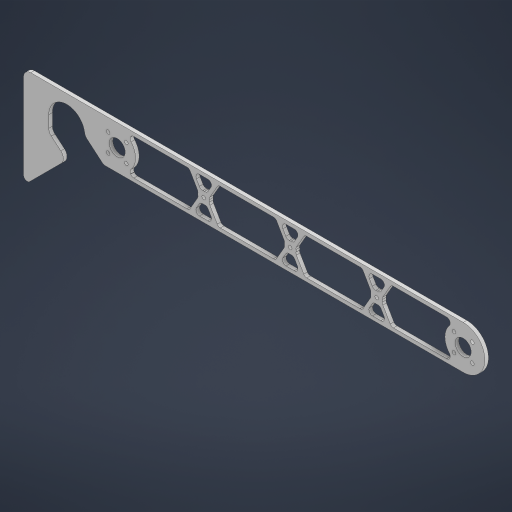
# Autodesk Inventor part: Arm1stLink
Saved by Autodesk Inventor 2023 (Build 270158000, 158)
## iProperties
Created: 2023-12-24
Part Number: Arm1stLink
Material: Generic
Document SubType Name: Modeling
Designer: kelle
Density: 1 g/cm^3
Appearance: Default
Author: kelle
Autodesk Inventor part; units mm, degrees
ref_plane "YZ Plane" through (0, 0, 0) normal (1, 0, 0) x (0, 1, 0)
ref_plane "XZ Plane" through (0, 0, 0) normal (0, 1, 0) x (-1, 0, 0)
ref_plane "XY Plane" through (0, 0, 0) normal (0, 0, 1) x (1, 0, 0)
sketch "Sketch1" plane through (0, 0, 0) normal (0, 0, 1) x (1, 0, 0)
  line L0 (152.4, 0) -> (-152.4, 0) construction
  line L1 (152.4, 19.05) -> (-152.4, 19.05)
  line L2 (-152.4, -19.05) -> (152.4, -19.05)
  arc A0 (152.4, -19.05) -> (152.4, 19.05) centre (152.4, 0) ccw
  arc A1 (-152.4, 19.05) -> (-152.4, -19.05) centre (-152.4, 0) ccw
  circle A2 centre (-152.4, 0) radius 7
  line L3 (-160.4, -8) -> (-144.4, -8) construction
  line L4 (-144.4, -8) -> (-144.4, 8) construction
  line L5 (-144.4, 8) -> (-160.4, 8) construction
  line L6 (-160.4, 8) -> (-160.4, -8) construction
  line L7 (-160.4, -8) -> (-144.4, 8) construction
  line L8 (-144.4, -8) -> (-160.4, 8) construction
  circle A3 centre (-160.4, 8) radius 1.5875
  circle A4 centre (-144.4, 8) radius 1.5875
  circle A5 centre (-160.4, -8) radius 1.5875
  circle A6 centre (-144.4, -8) radius 1.5875
  line L9 (0, 19.05) -> (0, -19.05) construction
  line L10 (-152.4, 0) -> (152.4, 0) construction
  circle A7 centre (152.4, 0) radius 7
  line L11 (160.4, -8) -> (144.4, -8) construction
  line L12 (144.4, -8) -> (144.4, 8) construction
  line L13 (144.4, 8) -> (160.4, 8) construction
  line L14 (160.4, 8) -> (160.4, -8) construction
  line L15 (160.4, -8) -> (144.4, 8) construction
  line L16 (144.4, -8) -> (160.4, 8) construction
  circle A8 centre (160.4, 8) radius 1.5875
  circle A9 centre (144.4, 8) radius 1.5875
  circle A10 centre (160.4, -8) radius 1.5875
  circle A11 centre (144.4, -8) radius 1.5875
  circle A12 centre (0, 0) radius 2
  circle A13 centre (-76.2, 0) radius 2
  circle A14 centre (76.2, 0) radius 2
  circle A15 centre (0, 0) radius 2
  dimension "d0" = 152.4
  dimension "d1" = 38.1
  dimension "d2" = 14
  dimension "d3" = 16
  dimension "d4" = 16
  dimension "d5" = 3.175
  dimension "d8" = 16
  dimension "d11" = 16
  dimension "d14" = 4
  dimension "d17" = 76.2
  dimension "d20" = 76.2
  constraints: 38 end point, 16 centre point, 11 symmetric about line, 5 coincident, 5 horizontal, 5 midpoint, 4 point on circle, 4 tangent, 3 parallel, 1 perpendicular, 1 vertical, 17 other
  measures "d0" distance of point (0, 0) L0.end
  measures "d1" diameter of A1
  measures "d2" diameter of A2
  measures "d3" distance of L5.end L4.end
  measures "d4" distance of L4.end L3.end
  measures "d5" diameter of A3
  measures "d8" distance of A3.centre A4.centre
  measures "d11" distance of A3.centre A5.centre
  measures "d14" diameter of A12
  measures "d17" distance of A12.centre A13.centre
  measures "d20" distance of A12.centre A14.centre
extrude "Extrusion1" add sketch "Sketch1" along normal blind 3.175
sketch "Sketch2" plane through (0, 0, 3.175) normal (0, 0, 1) x (1, 0, 0)
  arc A0 (-152.4, 19.05) -> (-152.4, -19.05) centre (-152.4, 0) ccw projected
  line L0 (-152.4, -19.05) -> (152.4, -19.05) projected
  arc A1 (152.4, -19.05) -> (152.4, 19.05) centre (152.4, 0) ccw projected
  line L1 (152.4, 19.05) -> (-152.4, 19.05) construction
  circle A2 centre (0, 0) radius 2 projected
  circle A3 centre (-76.2, 0) radius 2 projected
  circle A4 centre (76.2, 0) radius 2 projected
  circle A5 centre (160.4, -8) radius 1.5875 projected
  circle A6 centre (160.4, 8) radius 1.5875 projected
  circle A7 centre (152.4, 0) radius 7 projected
  circle A8 centre (144.4, -8) radius 1.5875 projected
  circle A9 centre (144.4, 8) radius 1.5875 projected
  circle A10 centre (-144.4, -8) radius 1.5875 projected
  circle A11 centre (-160.4, -8) radius 1.5875 projected
  circle A12 centre (-144.4, 8) radius 1.5875 projected
  circle A13 centre (-160.4, 8) radius 1.5875 projected
  circle A14 centre (-152.4, 0) radius 7 projected
  circle A15 centre (-152.4, 0) radius 12.9012 construction
  circle A16 centre (-152.4, 0) radius 16.0762
  arc A17 (-152.4, 15.875) -> (-152.4, -15.875) centre (-152.4, 0) ccw
  line L2 (-152.4, -15.875) -> (152.4, -15.875)
  arc A18 (152.4, -15.875) -> (152.4, 15.875) centre (152.4, 0) ccw
  line L3 (152.4, 15.875) -> (-152.4, 15.875)
  line L4 (-76.2, 19.05) -> (-76.2, -19.05) construction
  line L5 (-152.4, -19.05) -> (152.4, -19.05) construction
  line L6 (0, 19.05) -> (0, -19.05) construction
  circle A19 centre (152.4, 0) radius 16.0762
  circle A20 centre (-76.2, 0) radius 5.175
  circle A21 centre (0, 0) radius 5.175
  circle A22 centre (76.2, 0) radius 5.175
  line L7 (-152.4, 0) -> (-114.3, 0) construction
  line L8 (-152.4, 0) -> (-133.35, 32.9956)
  line L9 (-133.35, 32.9956) -> (-95.25, 32.9956)
  line L10 (-95.25, 32.9956) -> (-76.2, 0)
  line L11 (-76.2, 0) -> (-95.25, -32.9956)
  line L12 (-95.25, -32.9956) -> (-133.35, -32.9956)
  line L13 (-133.35, -32.9956) -> (-152.4, 0)
  line L14 (-97.0831, 29.8206) -> (-131.5169, 29.8206)
  line L15 (-131.5169, 29.8206) -> (-148.7338, 0)
  line L16 (-148.7338, 0) -> (-131.5169, -29.8206)
  line L17 (-131.5169, -29.8206) -> (-97.0831, -29.8206)
  line L18 (-97.0831, -29.8206) -> (-79.8662, 0)
  line L19 (-79.8662, 0) -> (-97.0831, 29.8206)
  line L20 (0, 0) -> (-19.05, 32.9956)
  line L21 (-57.15, 32.9956) -> (-76.2, 0)
  line L22 (-76.2, 0) -> (-57.15, -32.9956)
  line L23 (-19.05, -32.9956) -> (0, 0)
  line L24 (-20.8831, 29.8206) -> (-3.6662, 0)
  line L25 (-3.6662, 0) -> (-20.8831, -29.8206)
  line L26 (-55.3169, -29.8206) -> (-72.5338, 0)
  line L27 (-72.5338, 0) -> (-55.3169, 29.8206)
  line L28 (-152.4, 19.05) -> (152.4, 19.05)
  line L29 (152.4, 0) -> (133.35, 32.9956)
  line L30 (95.25, 32.9956) -> (76.2, 0)
  line L31 (76.2, 0) -> (95.25, -32.9956)
  line L32 (133.35, -32.9956) -> (152.4, 0)
  line L33 (131.5169, 29.8206) -> (148.7338, 0)
  line L34 (148.7338, 0) -> (131.5169, -29.8206)
  line L35 (97.0831, -29.8206) -> (79.8662, 0)
  line L36 (79.8662, 0) -> (97.0831, 29.8206)
  line L37 (20.8831, 29.8206) -> (3.6662, 0)
  line L38 (0, 0) -> (19.05, 32.9956)
  line L39 (19.05, -32.9956) -> (0, 0)
  line L40 (3.6662, 0) -> (20.8831, -29.8206)
  line L41 (55.3169, -29.8206) -> (72.5338, 0)
  line L42 (76.2, 0) -> (57.15, -32.9956)
  line L43 (72.5338, 0) -> (55.3169, 29.8206)
  line L44 (57.15, 32.9956) -> (76.2, 0)
  point P0 (141.7706, 12.0607)
  point P1 (139.5684, 15.875)
  point P2 (89.0316, 15.875)
  point P3 (80.9929, 1.9516)
  point P4 (80.9929, -1.9516)
  point P5 (89.0316, -15.875)
  point P6 (139.5684, -15.875)
  point P7 (141.7706, -12.0607)
  point P8 (85.3654, -15.875)
  point P9 (78.7875, -4.4817)
  point P10 (73.6125, -4.4817)
  point P11 (67.0346, -15.875)
  point P12 (78.7875, 4.4817)
  point P13 (85.3654, 15.875)
  point P14 (67.0346, 15.875)
  point P15 (73.6125, 4.4817)
  point P16 (12.8316, 15.875)
  point P17 (4.7929, 1.9516)
  point P18 (4.7929, -1.9516)
  point P19 (12.8316, -15.875)
  point P20 (63.3684, -15.875)
  point P21 (71.4071, -1.9516)
  point P22 (71.4071, 1.9516)
  point P23 (63.3684, 15.875)
  point P24 (9.1654, -15.875)
  point P25 (2.5875, -4.4817)
  point P26 (-2.5875, -4.4817)
  point P27 (-9.1654, -15.875)
  point P28 (2.5875, 4.4817)
  point P29 (9.1654, 15.875)
  point P30 (-9.1654, 15.875)
  point P31 (-2.5875, 4.4817)
  point P32 (-63.3684, 15.875)
  point P33 (-71.4071, 1.9516)
  point P34 (-71.4071, -1.9516)
  point P35 (-63.3684, -15.875)
  point P36 (-12.8316, -15.875)
  point P37 (-4.7929, -1.9516)
  point P38 (-4.7929, 1.9516)
  point P39 (-12.8316, 15.875)
  point P40 (-67.0346, -15.875)
  point P41 (-73.6125, -4.4817)
  point P42 (-78.7875, -4.4817)
  point P43 (-85.3654, -15.875)
  point P44 (-73.6125, 4.4817)
  point P45 (-67.0346, 15.875)
  point P46 (-85.3654, 15.875)
  point P47 (-78.7875, 4.4817)
  point P48 (-80.9929, 1.9516)
  point P49 (-89.0316, 15.875)
  point P50 (-139.5684, 15.875)
  point P51 (-141.7706, 12.0607)
  point P52 (-141.7706, -12.0607)
  point P53 (-139.5684, -15.875)
  point P54 (-89.0316, -15.875)
  point P55 (-80.9929, -1.9516)
  dimension "d25" = 3.175
  dimension "d26" = 3.175
  dimension "d27" = 3.175
  dimension "d28" = 3.175
  dimension "d29" = 3.175
  dimension "d30" = 38.1
  dimension "d31" = 3.175
  constraints: 84 end point, 36 symmetric about line, 8 centre point, 4 point on circle, 2 coincident, 2 midpoint, 2 point on line, 1 horizontal, 1 tangent, 1 vertical, 22 other
  measures "d25" radial gap between concentric circles of A15 A16
  measures "d26" distance between parallel lines of L1 L3
  measures "d27" radial gap between concentric circles of A3 A20
  measures "d28" radial gap between concentric circles of A2 A21
  measures "d29" radial gap between concentric circles of A4 A22
  measures "d30" distance of L7.start L7.end
  measures "d31" distance between parallel lines of L9 L14
extrude "Extrusion2" cut sketch "Sketch2" against normal through all contours L3 L19 A20 L18 L2 L16 A16 L15 | L3 L21 A20 L10 | L11 A20 L22 L2 | L3 L24 A21 L25 L2 L26 A20 L27 | L3 L38 A21 L20 | L23 A21 L39 L2 | L3 L43 A22 L41 L2 L40 A21 L37 | L3 L30 A22 L44 | L42 A22 L31 L2 | L3 L33 A19 L34 L2 L35 A22 L36
fillet "Fillet1" radius 3.175 56 edges at (-73.6125, -4.4817, 1.5875) (-67.0346, -15.875, 1.5875) (-78.7875, -4.4817, 1.5875) (-85.3654, -15.875, 1.5875) (2.5875, -4.4817, 1.5875) (9.1654, -15.875, 1.5875) (-2.5875, -4.4817, 1.5875) (-9.1654, -15.875, 1.5875) (-89.0316, 15.875, 1.5875) (-80.9929, 1.9516, 1.5875) (-139.5684, 15.875, 1.5875) (-141.7706, 12.0607, 1.5875) (-141.7706, -12.0607, 1.5875) (-139.5684, -15.875, 1.5875) (-89.0316, -15.875, 1.5875) (-80.9929, -1.9516, 1.5875) (78.7875, -4.4817, 1.5875) (85.3654, -15.875, 1.5875) (73.6125, -4.4817, 1.5875) (67.0346, -15.875, 1.5875) (4.7929, 1.9516, 1.5875) (12.8316, 15.875, 1.5875) (4.7929, -1.9516, 1.5875) (12.8316, -15.875, 1.5875) (63.3684, -15.875, 1.5875) (71.4071, -1.9516, 1.5875) (71.4071, 1.9516, 1.5875) (63.3684, 15.875, 1.5875) (139.5684, 15.875, 1.5875) (141.7706, 12.0607, 1.5875) (89.0316, 15.875, 1.5875) (80.9929, 1.9516, 1.5875) (80.9929, -1.9516, 1.5875) (89.0316, -15.875, 1.5875) (139.5684, -15.875, 1.5875) (141.7706, -12.0607, 1.5875) (-71.4071, 1.9516, 1.5875) (-63.3684, 15.875, 1.5875) (-71.4071, -1.9516, 1.5875) (-63.3684, -15.875, 1.5875) (-12.8316, -15.875, 1.5875) (-4.7929, -1.9516, 1.5875) (-4.7929, 1.9516, 1.5875) (-12.8316, 15.875, 1.5875) (-67.0346, 15.875, 1.5875) (-73.6125, 4.4817, 1.5875) (-85.3654, 15.875, 1.5875) (-78.7875, 4.4817, 1.5875) (9.1654, 15.875, 1.5875) (2.5875, 4.4817, 1.5875) (-9.1654, 15.875, 1.5875) (-2.5875, 4.4817, 1.5875) (85.3654, 15.875, 1.5875) (78.7875, 4.4817, 1.5875) (67.0346, 15.875, 1.5875) (73.6125, 4.4817, 1.5875)
sketch "Sketch3" plane through (0, 0, 3.175) normal (0, 0, 1) x (1, 0, 0)
  line L0 (-82.6158, -11.1125) -> (-80.0614, -6.6882) projected
  arc A0 (-76.889, -5.1289) -> (-80.0614, -6.6882) centre (-77.3118, -8.2757) ccw projected
  arc A1 (-76.889, -5.1289) -> (-75.511, -5.1289) centre (-76.2, 0) ccw projected
  arc A2 (-72.3386, -6.6882) -> (-75.511, -5.1289) centre (-75.0882, -8.2757) ccw projected
  line L1 (-72.3386, -6.6882) -> (-69.7842, -11.1125) projected
  arc A3 (-72.5338, -15.875) -> (-69.7842, -11.1125) centre (-72.5338, -12.7) ccw projected
  line L2 (-72.5338, -15.875) -> (-79.8662, -15.875) projected
  arc A4 (-82.6158, -11.1125) -> (-79.8662, -15.875) centre (-79.8662, -12.7) ccw projected
  line L3 (11.9151, -14.2875) -> (5.4607, -3.1082) projected
  arc A5 (5.0885, -0.9425) -> (5.4607, -3.1082) centre (8.2103, -1.5207) ccw projected
  arc A6 (5.0885, -0.9425) -> (5.0885, 0.9425) centre (0, 0) ccw projected
  arc A7 (5.4607, 3.1082) -> (5.0885, 0.9425) centre (8.2103, 1.5207) ccw projected
  line L4 (5.4607, 3.1082) -> (11.9151, 14.2875) projected
  arc A8 (14.6647, 15.875) -> (11.9151, 14.2875) centre (14.6647, 12.7) ccw projected
  line L5 (14.6647, 15.875) -> (61.5353, 15.875) projected
  arc A9 (64.2849, 14.2875) -> (61.5353, 15.875) centre (61.5353, 12.7) ccw projected
  line L6 (64.2849, 14.2875) -> (70.7393, 3.1082) projected
  arc A10 (71.1115, 0.9425) -> (70.7393, 3.1082) centre (67.9897, 1.5207) ccw projected
  arc A11 (71.1115, 0.9425) -> (71.1115, -0.9425) centre (76.2, 0) ccw projected
  arc A12 (70.7393, -3.1082) -> (71.1115, -0.9425) centre (67.9897, -1.5207) ccw projected
  line L7 (70.7393, -3.1082) -> (64.2849, -14.2875) projected
  arc A13 (61.5353, -15.875) -> (64.2849, -14.2875) centre (61.5353, -12.7) ccw projected
  line L8 (61.5353, -15.875) -> (14.6647, -15.875) projected
  arc A14 (11.9151, -14.2875) -> (14.6647, -15.875) centre (14.6647, -12.7) ccw projected
  line L9 (81.6607, 3.1082) -> (88.1151, 14.2875) projected
  arc A15 (90.8647, 15.875) -> (88.1151, 14.2875) centre (90.8647, 12.7) ccw projected
  line L10 (90.8647, 15.875) -> (137.7353, 15.875) projected
  arc A16 (140.4849, 14.2875) -> (137.7353, 15.875) centre (137.7353, 12.7) ccw projected
  line L11 (140.4849, 14.2875) -> (140.5635, 14.1515) projected
  arc A17 (140.2195, 10.4919) -> (140.5635, 14.1515) centre (137.8138, 12.564) ccw projected
  arc A18 (140.2195, 10.4919) -> (140.2195, -10.4919) centre (152.4, 0) ccw projected
  arc A19 (140.5635, -14.1515) -> (140.2195, -10.4919) centre (137.8138, -12.564) ccw projected
  line L12 (140.5635, -14.1515) -> (140.4849, -14.2875) projected
  arc A20 (137.7353, -15.875) -> (140.4849, -14.2875) centre (137.7353, -12.7) ccw projected
  line L13 (137.7353, -15.875) -> (90.8647, -15.875) projected
  arc A21 (88.1151, -14.2875) -> (90.8647, -15.875) centre (90.8647, -12.7) ccw projected
  line L14 (88.1151, -14.2875) -> (81.6607, -3.1082) projected
  arc A22 (81.2885, -0.9425) -> (81.6607, -3.1082) centre (84.4103, -1.5207) ccw projected
  arc A23 (81.2885, -0.9425) -> (81.2885, 0.9425) centre (76.2, 0) ccw projected
  arc A24 (81.6607, 3.1082) -> (81.2885, 0.9425) centre (84.4103, 1.5207) ccw projected
  line L15 (-6.4158, -11.1125) -> (-3.8614, -6.6882) projected
  arc A25 (-0.689, -5.1289) -> (-3.8614, -6.6882) centre (-1.1118, -8.2757) ccw projected
  arc A26 (-0.689, -5.1289) -> (0.689, -5.1289) centre (0, 0) ccw projected
  arc A27 (3.8614, -6.6882) -> (0.689, -5.1289) centre (1.1118, -8.2757) ccw projected
  line L16 (3.8614, -6.6882) -> (6.4158, -11.1125) projected
  arc A28 (3.6662, -15.875) -> (6.4158, -11.1125) centre (3.6662, -12.7) ccw projected
  line L17 (3.6662, -15.875) -> (-3.6662, -15.875) projected
  arc A29 (-6.4158, -11.1125) -> (-3.6662, -15.875) centre (-3.6662, -12.7) ccw projected
  line L18 (-80.0614, 6.6882) -> (-82.6158, 11.1125) projected
  arc A30 (-79.8662, 15.875) -> (-82.6158, 11.1125) centre (-79.8662, 12.7) ccw projected
  line L19 (-79.8662, 15.875) -> (-72.5338, 15.875) projected
  arc A31 (-69.7842, 11.1125) -> (-72.5338, 15.875) centre (-72.5338, 12.7) ccw projected
  line L20 (-69.7842, 11.1125) -> (-72.3386, 6.6882) projected
  arc A32 (-75.511, 5.1289) -> (-72.3386, 6.6882) centre (-75.0882, 8.2757) ccw projected
  arc A33 (-75.511, 5.1289) -> (-76.889, 5.1289) centre (-76.2, 0) ccw projected
  arc A34 (-80.0614, 6.6882) -> (-76.889, 5.1289) centre (-77.3118, 8.2757) ccw projected
  line L21 (-64.2849, -14.2875) -> (-70.7393, -3.1082) projected
  arc A35 (-71.1115, -0.9425) -> (-70.7393, -3.1082) centre (-67.9897, -1.5207) ccw projected
  arc A36 (-71.1115, -0.9425) -> (-71.1115, 0.9425) centre (-76.2, 0) ccw projected
  arc A37 (-70.7393, 3.1082) -> (-71.1115, 0.9425) centre (-67.9897, 1.5207) ccw projected
  line L22 (-70.7393, 3.1082) -> (-64.2849, 14.2875) projected
  arc A38 (-61.5353, 15.875) -> (-64.2849, 14.2875) centre (-61.5353, 12.7) ccw projected
  line L23 (-61.5353, 15.875) -> (-14.6647, 15.875) projected
  arc A39 (-11.9151, 14.2875) -> (-14.6647, 15.875) centre (-14.6647, 12.7) ccw projected
  line L24 (-11.9151, 14.2875) -> (-5.4607, 3.1082) projected
  arc A40 (-5.0885, 0.9425) -> (-5.4607, 3.1082) centre (-8.2103, 1.5207) ccw projected
  arc A41 (-5.0885, 0.9425) -> (-5.0885, -0.9425) centre (0, 0) ccw projected
  arc A42 (-5.4607, -3.1082) -> (-5.0885, -0.9425) centre (-8.2103, -1.5207) ccw projected
  line L25 (-5.4607, -3.1082) -> (-11.9151, -14.2875) projected
  arc A43 (-14.6647, -15.875) -> (-11.9151, -14.2875) centre (-14.6647, -12.7) ccw projected
  line L26 (-14.6647, -15.875) -> (-61.5353, -15.875) projected
  arc A44 (-64.2849, -14.2875) -> (-61.5353, -15.875) centre (-61.5353, -12.7) ccw projected
  line L27 (72.3386, 6.6882) -> (69.7842, 11.1125) projected
  arc A45 (72.5338, 15.875) -> (69.7842, 11.1125) centre (72.5338, 12.7) ccw projected
  line L28 (72.5338, 15.875) -> (79.8662, 15.875) projected
  arc A46 (82.6158, 11.1125) -> (79.8662, 15.875) centre (79.8662, 12.7) ccw projected
  line L29 (82.6158, 11.1125) -> (80.0614, 6.6882) projected
  arc A47 (76.889, 5.1289) -> (80.0614, 6.6882) centre (77.3118, 8.2757) ccw projected
  arc A48 (76.889, 5.1289) -> (75.511, 5.1289) centre (76.2, 0) ccw projected
  arc A49 (72.3386, 6.6882) -> (75.511, 5.1289) centre (75.0882, 8.2757) ccw projected
  line L30 (69.7842, -11.1125) -> (72.3386, -6.6882) projected
  arc A50 (75.511, -5.1289) -> (72.3386, -6.6882) centre (75.0882, -8.2757) ccw projected
  arc A51 (75.511, -5.1289) -> (76.889, -5.1289) centre (76.2, 0) ccw projected
  arc A52 (80.0614, -6.6882) -> (76.889, -5.1289) centre (77.3118, -8.2757) ccw projected
  line L31 (80.0614, -6.6882) -> (82.6158, -11.1125) projected
  arc A53 (79.8662, -15.875) -> (82.6158, -11.1125) centre (79.8662, -12.7) ccw projected
  line L32 (79.8662, -15.875) -> (72.5338, -15.875) projected
  arc A54 (69.7842, -11.1125) -> (72.5338, -15.875) centre (72.5338, -12.7) ccw projected
  line L33 (-3.8614, 6.6882) -> (-6.4158, 11.1125) projected
  arc A55 (-3.6662, 15.875) -> (-6.4158, 11.1125) centre (-3.6662, 12.7) ccw projected
  line L34 (-3.6662, 15.875) -> (3.6662, 15.875) projected
  arc A56 (6.4158, 11.1125) -> (3.6662, 15.875) centre (3.6662, 12.7) ccw projected
  line L35 (6.4158, 11.1125) -> (3.8614, 6.6882) projected
  arc A57 (0.689, 5.1289) -> (3.8614, 6.6882) centre (1.1118, 8.2757) ccw projected
  arc A58 (0.689, 5.1289) -> (-0.689, 5.1289) centre (0, 0) ccw projected
  arc A59 (-3.8614, 6.6882) -> (-0.689, 5.1289) centre (-1.1118, 8.2757) ccw projected
  line L36 (-140.5635, 14.1515) -> (-140.4849, 14.2875) projected
  arc A60 (-137.7353, 15.875) -> (-140.4849, 14.2875) centre (-137.7353, 12.7) ccw projected
  line L37 (-137.7353, 15.875) -> (-90.8647, 15.875) projected
  arc A61 (-88.1151, 14.2875) -> (-90.8647, 15.875) centre (-90.8647, 12.7) ccw projected
  line L38 (-88.1151, 14.2875) -> (-81.6607, 3.1082) projected
  arc A62 (-81.2885, 0.9425) -> (-81.6607, 3.1082) centre (-84.4103, 1.5207) ccw projected
  arc A63 (-81.2885, 0.9425) -> (-81.2885, -0.9425) centre (-76.2, 0) ccw projected
  arc A64 (-81.6607, -3.1082) -> (-81.2885, -0.9425) centre (-84.4103, -1.5207) ccw projected
  line L39 (-81.6607, -3.1082) -> (-88.1151, -14.2875) projected
  arc A65 (-90.8647, -15.875) -> (-88.1151, -14.2875) centre (-90.8647, -12.7) ccw projected
  line L40 (-90.8647, -15.875) -> (-137.7353, -15.875) projected
  arc A66 (-140.4849, -14.2875) -> (-137.7353, -15.875) centre (-137.7353, -12.7) ccw projected
  line L41 (-140.4849, -14.2875) -> (-140.5635, -14.1515) projected
  arc A67 (-140.2195, -10.4919) -> (-140.5635, -14.1515) centre (-137.8138, -12.564) ccw projected
  arc A68 (-140.2195, -10.4919) -> (-140.2195, 10.4919) centre (-152.4, 0) ccw projected
  arc A69 (-140.5635, 14.1515) -> (-140.2195, 10.4919) centre (-137.8138, 12.564) ccw projected
  arc A70 (-152.4, 19.05) -> (-152.4, -19.05) centre (-152.4, 0) ccw projected
  line L42 (-152.4, -19.05) -> (152.4, -19.05) projected
  arc A71 (152.4, -19.05) -> (152.4, 19.05) centre (152.4, 0) ccw projected
  line L43 (152.4, 19.05) -> (-152.4, 19.05) projected
  circle A72 centre (0, 0) radius 2 projected
  circle A73 centre (-76.2, 0) radius 2 projected
  circle A74 centre (76.2, 0) radius 2 projected
  circle A75 centre (160.4, -8) radius 1.5875 projected
  circle A76 centre (160.4, 8) radius 1.5875 projected
  circle A77 centre (152.4, 0) radius 7 projected
  circle A78 centre (144.4, -8) radius 1.5875 projected
  circle A79 centre (144.4, 8) radius 1.5875 projected
  circle A80 centre (-144.4, -8) radius 1.5875 projected
  circle A81 centre (-160.4, -8) radius 1.5875 projected
  circle A82 centre (-144.4, 8) radius 1.5875 projected
  circle A83 centre (-160.4, 8) radius 1.5875 projected
  circle A84 centre (-152.4, 0) radius 7 projected
  circle A85 centre (-76.2, 0) radius 2 projected
  circle A86 centre (-76.2, 0) radius 1.5875
  circle A87 centre (0, 0) radius 2 projected
  circle A88 centre (0, 0) radius 1.5875
  circle A89 centre (76.2, 0) radius 2 projected
  circle A90 centre (76.2, 0) radius 1.5875
  dimension "d35" = 3.175
  dimension "d36" = 3.175
  dimension "d37" = 3.175
  constraints: 3 centre point, 3 coincident
  measures "d35" diameter of A86
  measures "d36" diameter of A88
  measures "d37" diameter of A90
extrude "Extrusion3" add sketch "Sketch3" against normal blind 3.175 contours A72 | A73 | A74
sketch "Sketch4" plane through (0, 0, 3.175) normal (0, 0, 1) x (1, 0, 0)
  line L0 (152.4, 19.05) -> (-152.4, 19.05) projected
  line L1 (-152.4, 19.05) -> (-234.95, 19.05)
  line L2 (-234.95, 19.05) -> (-234.95, -19.05)
  line L3 (-234.95, -19.05) -> (-152.4, -19.05)
  line L4 (-152.4, -19.05) -> (-152.4, 19.05)
  line L5 (-234.95, 19.05) -> (-196.85, 19.05)
  line L6 (-196.85, 19.05) -> (-196.85, -69.85)
  line L7 (-196.85, -69.85) -> (-234.95, -69.85)
  line L8 (-234.95, -69.85) -> (-234.95, 19.05)
  line L9 (-234.95, -69.85) -> (-196.85, -31.75)
  circle A0 centre (-196.85, -5.0447) radius 15.875
  line L10 (-164.4274, -19.05) -> (-180.975, -5.0447)
  line L11 (-212.725, 0) -> (-212.725, -19.05)
  line L12 (-196.85, -31.75) -> (-212.725, -18.314)
  circle A1 centre (-152.4, 0) radius 7 projected
  circle A2 centre (-144.4, -8) radius 1.5875 projected
  circle A3 centre (-144.4, 8) radius 1.5875 projected
  circle A4 centre (-160.4, 8) radius 1.5875 projected
  circle A5 centre (-160.4, -8) radius 1.5875 projected
  point P0 (0, 0)
  point P1 (-211.8554, -19.05)
  point P2 (-212.725, -5.0447)
  point P3 (-152.4, -7)
  point P4 (-152.4, 7)
  dimension "d45" = 31.75
  dimension "d40" = 82.55
  dimension "d41" = 38.1
  dimension "d42" = 38.1
  dimension "d43" = 88.9
  dimension "d44" = 45
  constraints: 24 end point, 5 parallel, 5 point on line, 3 perpendicular, 2 horizontal, 1 vertical, 3 other
  measures "d40" distance of L3.end L2.end
  measures "d41" distance of L2.end L1.end
  measures "d42" distance of L6.end L7.end
  measures "d43" distance of L5.end L6.end
  measures "d44" angle of L7 L9
extrude "Extrusion4" add sketch "Sketch4" against normal blind 3.175 contours L4 A1 L3 L10 A0 L6 L1 | L6 A0 L11 L3 L2 L1 | L3 L12 L9 L8
fillet "Fillet2" radius 6.35 3 edges at (-211.8554, -19.05, 1.5875) (-212.725, -19.05, 1.5875) (-196.85, -31.75, 1.5875)
fillet "Fillet3" radius 6.35 2 edges at (-180.975, -5.0447, 1.5875) (-234.95, 19.05, 1.5875)
fillet "Fillet4" radius 3.175 2 edges at (-164.4274, -19.05, 1.5875) (-234.95, -69.85, 1.5875)
body "Solid1"
